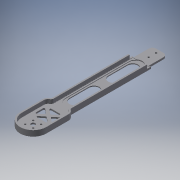
# Autodesk Inventor part: Arm
Saved by Autodesk Inventor 2016 (Build 200138000, 138)
## iProperties
Created: 2015-04-14
Part Number: Arm
Material: Generic
Document SubType Name: Modeling
Designer: Vasanth
Density: 1 g/cm^3
Appearance: Default
Author: Vasanth
Autodesk Inventor part; units mm, degrees
ref_plane "YZ Plane" through (0, 0, 0) normal (1, 0, 0) x (0, 1, 0)
ref_plane "XZ Plane" through (0, 0, 0) normal (0, 1, 0) x (-1, 0, 0)
ref_plane "XY Plane" through (0, 0, 0) normal (0, 0, 1) x (1, 0, 0)
sketch "Sketch1" plane through (0, 0, 0) normal (0, 1, 0) x (-1, 0, 0)
  line L0 (52.0335, 19.2292) -> (51.733, 19.2292)
  line L1 (38.3582, 166.9806) -> (38.3582, 31.0212)
  line L2 (6.6082, 166.9806) -> (6.6082, 31.0212)
  line L3 (38.3582, 31.0212) -> (35.1832, 32.9161)
  line L4 (35.1832, 32.9161) -> (35.1832, 6.5292)
  line L5 (9.7832, 32.9161) -> (9.7832, 6.5292)
  line L6 (16.1332, 0.1792) -> (28.8332, 0.1792)
  line L7 (44.7082, 216.0792) -> (44.7082, 177.9792)
  line L8 (0.2582, 177.9792) -> (0.2582, 216.0792)
  arc A0 (44.7082, 216.0792) -> (0.2582, 216.0792) centre (22.4832, 216.0792) ccw
  arc A1 (39.9457, 169.7303) -> (38.3582, 166.9806) centre (41.5332, 166.9806) ccw
  arc A2 (28.8332, 0.1792) -> (35.1832, 6.5292) centre (28.8332, 6.5292) ccw
  arc A3 (9.7832, 6.5292) -> (16.1332, 0.1792) centre (16.1332, 6.5292) ccw
  arc A4 (39.9457, 169.7303) -> (44.7082, 177.9792) centre (35.1832, 177.9792) ccw
  arc A5 (0.2582, 177.9792) -> (5.0207, 169.7303) centre (9.7832, 177.9792) ccw
  arc A6 (6.6082, 166.9806) -> (5.0207, 169.7303) centre (3.4332, 166.9806) ccw
  line L9 (9.7832, 32.9161) -> (6.6082, 31.0212)
  constraints: 20 end point, 15 tangent, 14 point on circle, 7 centre point, 4 vertical, 3 equal radius, 3 parallel, 1 horizontal
extrude "Extrusion1" add sketch "Sketch1" along normal blind 9.525
sketch "Sketch5" plane through (0, 9.525, 0) normal (0, 1, 0) x (1, 0, 0)
  line L0 (-52.0335, -19.2292) -> (-51.733, -19.2292)
  line L1 (-35.1832, -32.9161) -> (-35.1832, -34.2351)
  line L2 (-9.7832, -32.9161) -> (-9.7832, -34.2351)
  line L3 (-2.7995, -216.0792) -> (-2.7995, -177.9792)
  line L4 (-42.167, -216.0792) -> (-42.167, -177.9792)
  line L5 (-9.1495, -166.9806) -> (-9.1495, -34.2351)
  line L6 (-9.1495, -34.2351) -> (-9.7832, -34.2351)
  line L7 (-35.1832, -34.2351) -> (-35.9386, -34.2351)
  line L8 (-35.1832, -6.5292) -> (-35.1832, -32.9161)
  line L9 (-35.1832, -32.9161) -> (-35.1832, -6.5292) projected
  line L10 (-9.7832, -32.9161) -> (-9.7832, -6.5292)
  arc A0 (-9.7832, -6.5292) -> (-16.1332, -0.1792) centre (-16.1332, -6.5292) ccw
  arc A1 (-28.8332, -0.1792) -> (-35.1832, -6.5292) centre (-28.8332, -6.5292) ccw
  arc A2 (-38.6751, -171.9311) -> (-42.167, -177.9792) centre (-35.1832, -177.9792) ccw
  arc A3 (-2.7995, -177.9792) -> (-6.2914, -171.9311) centre (-9.7832, -177.9792) ccw
  arc A4 (-9.1495, -166.9806) -> (-6.2914, -171.9311) centre (-3.4332, -166.9806) ccw
  arc A5 (-38.6751, -171.9311) -> (-35.9386, -168.1538) centre (-41.5332, -166.9806) ccw
  line L11 (-28.8332, -0.1792) -> (-16.1332, -0.1792)
  arc A6 (-9.7832, -6.5292) -> (-16.1332, -0.1792) centre (-16.1332, -6.5292) ccw projected
  line L12 (-16.1332, -0.1792) -> (-28.8332, -0.1792) projected
  arc A7 (-42.167, -216.0792) -> (-2.7995, -216.0792) centre (-22.4832, -216.0792) ccw
  line L13 (-35.9386, -34.2351) -> (-35.9386, -168.1538)
  line L14 (-38.3582, -166.9806) -> (-38.3582, -31.0212) projected
  constraints: 24 end point, 14 point on circle, 7 centre point, 3 vertical, 2 collinear, 2 parallel, 1 horizontal, 1 point on line, 1 tangent
extrude "Extrusion2" cut sketch "Sketch5" against normal blind 6.35
sketch "Sketch6" plane through (0, 9.525, 0) normal (0, 1, 0) x (1, 0, 0)
  circle A0 centre (-22.4832, -19.2292) radius 1.5001
  circle A1 centre (-22.4832, -6.5292) radius 1.5001
  line L0 (-13.5932, -145.3906) -> (-13.5932, -112.3706)
  line L1 (-31.3732, -145.3906) -> (-31.3732, -112.3706)
  line L2 (-31.3732, -79.3506) -> (-31.3732, -46.3306)
  line L3 (-13.5932, -79.3506) -> (-13.5932, -46.3306)
  arc A2 (-13.5932, -112.3706) -> (-31.3732, -112.3706) centre (-22.4832, -112.3706) ccw
  arc A3 (-31.3732, -145.3906) -> (-13.5932, -145.3906) centre (-22.4832, -145.3906) ccw
  arc A4 (-31.3732, -79.3506) -> (-13.5932, -79.3506) centre (-22.4832, -79.3506) ccw
  arc A5 (-13.5932, -46.3306) -> (-31.3732, -46.3306) centre (-22.4832, -46.3306) ccw
  line L4 (-149.0334, -127.8705) -> (-176.2084, -108.4598)
  line L5 (-109.1652, -138.2049) -> (-81.9901, -157.6157)
  line L6 (-123.9321, -113.1036) -> (-104.5213, -85.9286)
  line L7 (-109.6885, -190.1877) -> (-148.51, -190.1877)
  line L8 (-109.6885, -75.8877) -> (-148.51, -75.8877)
  arc A6 (-148.51, -75.8877) -> (-153.6772, -85.9286) centre (-148.51, -82.2377) ccw
  circle A7 centre (-82.019, -85.9575) radius 1.5001
  circle A8 centre (-176.1795, -180.118) radius 1.5001
  circle A9 centre (-176.1795, -85.9575) radius 1.5001
  circle A10 centre (-151.5993, -155.5378) radius 1.5001
  circle A11 centre (-106.5992, -155.5378) radius 1.5001
  circle A12 centre (-106.5992, -110.5377) radius 1.5001
  circle A13 centre (-151.5993, -110.5377) radius 1.5001
  circle A14 centre (-16.8264, -221.736) radius 1.5001
  circle A15 centre (-29.2008, -222.7967) radius 1.5001
  circle A16 centre (-15.7656, -209.3616) radius 1.5001
  line L9 (-149.0334, -138.2049) -> (-176.2084, -157.6157)
  line L10 (-134.2665, -152.9718) -> (-153.6772, -180.1469)
  line L11 (-109.1652, -127.8705) -> (-81.9901, -108.4598)
  line L12 (-134.2665, -113.1036) -> (-153.6772, -85.9286)
  line L13 (-186.2493, -113.627) -> (-186.2493, -152.4485)
  line L14 (-71.9493, -152.4485) -> (-71.9493, -113.627)
  arc A17 (-104.5213, -85.9286) -> (-109.6885, -75.8877) centre (-109.6885, -82.2377) ccw
  arc A18 (-134.2665, -113.1036) -> (-123.9321, -113.1036) centre (-129.0993, -109.4128) ccw
  arc A19 (-149.0334, -138.2049) -> (-149.0334, -127.8705) centre (-152.7242, -133.0377) ccw
  arc A20 (-186.2493, -152.4485) -> (-176.2084, -157.6157) centre (-179.8993, -152.4485) ccw
  arc A21 (-176.2084, -108.4598) -> (-186.2493, -113.627) centre (-179.8993, -113.627) ccw
  arc A22 (-153.6772, -180.1469) -> (-148.51, -190.1877) centre (-148.51, -183.8377) ccw
  arc A23 (-123.9321, -152.9718) -> (-134.2665, -152.9718) centre (-129.0993, -156.6627) ccw
  arc A24 (-81.9901, -157.6157) -> (-71.9493, -152.4485) centre (-78.2993, -152.4485) ccw
  arc A25 (-71.9493, -113.627) -> (-81.9901, -108.4598) centre (-78.2993, -113.627) ccw
  arc A26 (-109.1652, -127.8705) -> (-109.1652, -138.2049) centre (-105.4743, -133.0377) ccw
  arc A27 (-127.8075, -223.1112) -> (-130.3911, -223.1112) centre (-129.0993, -224.034) ccw
  line L15 (-134.0828, -216.8359) -> (-140.8766, -211.9832)
  line L16 (-134.0828, -219.4195) -> (-140.8766, -224.2722)
  line L17 (-127.8075, -223.1112) -> (-122.9548, -229.905)
  line L18 (-130.3911, -223.1112) -> (-135.2438, -229.905)
  line L19 (-124.1158, -219.4195) -> (-117.322, -224.2722)
  line L20 (-124.1158, -216.8359) -> (-117.322, -211.9832)
  line L21 (-127.8075, -213.1442) -> (-122.9548, -206.3504)
  line L22 (-130.3911, -213.1442) -> (-135.2437, -206.3504)
  arc A28 (-130.3911, -213.1442) -> (-127.8075, -213.1442) centre (-129.0993, -212.2215) ccw
  arc A29 (-134.0828, -219.4195) -> (-134.0828, -216.8359) centre (-135.0055, -218.1277) ccw
  arc A30 (-124.1158, -216.8359) -> (-124.1158, -219.4195) centre (-123.193, -218.1277) ccw
  line L23 (-117.322, -224.2722) -> (-108.7122, -230.3009)
  line L24 (-117.322, -211.9832) -> (-108.7122, -205.9546)
  line L25 (-135.2438, -229.905) -> (-137.004, -232.4188)
  line L26 (-122.9548, -229.905) -> (-121.1946, -232.4188)
  line L27 (-123.2752, -236.4157) -> (-134.9233, -236.4157)
  line L28 (-123.24, -199.8397) -> (-134.9586, -199.8397)
  line L29 (-153.4832, -207.9142) -> (-153.4832, -228.3413)
  line L30 (-104.7153, -228.2202) -> (-104.7153, -208.0352)
  line L31 (-140.8766, -211.9832) -> (-149.4669, -205.8473)
  line L32 (-140.8766, -224.2722) -> (-149.4669, -230.4082)
  line L33 (-122.9548, -206.3504) -> (-121.1731, -203.8561)
  line L34 (-135.2437, -206.3504) -> (-137.0254, -203.8561)
  arc A31 (-108.7122, -230.3009) -> (-104.7153, -228.2202) centre (-107.2553, -228.2202) ccw
  arc A32 (-104.7153, -208.0352) -> (-108.7122, -205.9546) centre (-107.2553, -208.0352) ccw
  arc A33 (-121.1731, -203.8561) -> (-123.24, -199.8397) centre (-123.24, -202.3797) ccw
  arc A34 (-134.9586, -199.8397) -> (-137.0254, -203.8561) centre (-134.9586, -202.3797) ccw
  arc A35 (-149.4669, -205.8473) -> (-153.4832, -207.9142) centre (-150.9432, -207.9142) ccw
  arc A36 (-153.4832, -228.3413) -> (-149.4669, -230.4082) centre (-150.9432, -228.3413) ccw
  arc A37 (-137.004, -232.4188) -> (-134.9233, -236.4157) centre (-134.9233, -233.8757) ccw
  arc A38 (-123.2752, -236.4157) -> (-121.1946, -232.4188) centre (-123.2752, -233.8757) ccw
  arc A39 (-109.6885, -190.1877) -> (-104.5213, -180.1469) centre (-109.6885, -183.8377) ccw
  line L35 (-123.9321, -152.9718) -> (-104.5213, -180.1469)
  circle A40 centre (-82.019, -180.118) radius 1.5001
  circle A41 centre (-22.4832, -216.0792) radius 3.5001
  circle A42 centre (-28.1401, -210.4223) radius 1.5001
  arc A43 (-92.1218, -170.0152) -> (-89.8767, -172.2603) centre (-90.9993, -171.1377) ccw
  arc A44 (-82.019, -169.0055) -> (-82.019, -165.8305) centre (-82.019, -167.418) ccw
  arc A45 (-82.019, -169.0055) -> (-89.8767, -172.2603) centre (-82.019, -180.118) ccw
  arc A46 (-82.019, -165.8305) -> (-92.1218, -170.0152) centre (-82.019, -180.118) ccw
  arc A47 (-82.019, -100.245) -> (-82.019, -97.07) centre (-82.019, -98.6575) ccw
  arc A48 (-92.1218, -96.0603) -> (-82.019, -100.245) centre (-82.019, -85.9575) ccw
  arc A49 (-89.8767, -93.8152) -> (-82.019, -97.07) centre (-82.019, -85.9575) ccw
  arc A50 (-89.8767, -93.8152) -> (-92.1218, -96.0603) centre (-90.9993, -94.9377) ccw
  arc A51 (-176.1795, -165.8305) -> (-176.1795, -169.0055) centre (-176.1795, -167.418) ccw
  arc A52 (-166.0767, -170.0152) -> (-176.1795, -165.8305) centre (-176.1795, -180.118) ccw
  arc A53 (-168.3218, -172.2603) -> (-176.1795, -169.0055) centre (-176.1795, -180.118) ccw
  arc A54 (-168.3218, -172.2603) -> (-166.0767, -170.0152) centre (-167.1993, -171.1377) ccw
  arc A55 (-176.1795, -97.07) -> (-176.1795, -100.245) centre (-176.1795, -98.6575) ccw
  arc A56 (-176.1795, -100.245) -> (-166.0767, -96.0603) centre (-176.1795, -85.9575) ccw
  arc A57 (-176.1795, -97.07) -> (-168.3218, -93.8152) centre (-176.1795, -85.9575) ccw
  arc A58 (-166.0767, -96.0603) -> (-168.3218, -93.8152) centre (-167.1993, -94.9377) ccw
  arc A59 (-15.4908, -202.4266) -> (-14.4897, -199.6071) centre (-15.4908, -200.8391) ccw
  arc A60 (-30.4768, -199.6071) -> (-29.4757, -202.4266) centre (-29.4757, -200.8391) ccw
  arc A61 (-21.4822, -193.9257) -> (-23.4843, -193.9257) centre (-22.4832, -195.1578) ccw
  arc A62 (-17.1906, -188.8121) -> (-17.1906, -191.2762) centre (-16.1895, -190.0442) ccw
  arc A63 (-7.2432, -184.0651) -> (-9.8318, -182.833) centre (-8.8307, -184.0651) ccw
  arc A64 (-9.8318, -197.2553) -> (-7.2432, -196.0232) centre (-8.8307, -196.0232) ccw
  arc A65 (-14.4897, -180.4812) -> (-15.4908, -177.6617) centre (-15.4908, -179.2492) ccw
  arc A66 (-29.4757, -177.6617) -> (-30.4768, -180.4812) centre (-29.4757, -179.2492) ccw
  arc A67 (-23.4843, -186.1626) -> (-21.4822, -186.1626) centre (-22.4832, -184.9305) ccw
  arc A68 (-27.7758, -191.2762) -> (-27.7758, -188.8121) centre (-28.7769, -190.0442) ccw
  arc A69 (-37.7232, -196.0232) -> (-35.1347, -197.2553) centre (-36.1357, -196.0232) ccw
  arc A70 (-35.1347, -182.833) -> (-37.7232, -184.0651) centre (-36.1357, -184.0651) ccw
  line L36 (-15.4908, -202.4266) -> (-29.4757, -202.4266)
  line L37 (-14.4897, -199.6071) -> (-21.4822, -193.9257)
  line L38 (-23.4843, -193.9257) -> (-30.4768, -199.6071)
  line L39 (-35.1347, -197.2553) -> (-27.7758, -191.2762)
  line L40 (-27.7758, -188.8121) -> (-35.1347, -182.833)
  line L41 (-37.7232, -184.0651) -> (-37.7232, -196.0232)
  line L42 (-30.4768, -180.4812) -> (-23.4843, -186.1626)
  line L43 (-21.4822, -186.1626) -> (-14.4897, -180.4812)
  line L44 (-15.4908, -177.6617) -> (-29.4757, -177.6617)
  line L45 (-7.2432, -196.0232) -> (-7.2432, -184.0651)
  line L46 (-9.8318, -182.833) -> (-17.1906, -188.8121)
  line L47 (-17.1906, -191.2762) -> (-9.8318, -197.2553)
  point P0 (0, 0)
  constraints: 112 point on circle, 99 tangent, 96 end point, 71 centre point, 49 equal radius, 10 parallel, 10 perpendicular, 8 concentric, 2 collinear
extrude "Extrusion3" cut sketch "Sketch6" against normal blind 25.4
sketch "Sketch7" plane through (0, 9.525, 0) normal (0, 1, 0) x (1, 0, 0)
  line L0 (-52.0335, -19.2292) -> (-51.733, -19.2292)
  line L1 (0, -16.7662) -> (-44.6659, -16.7662)
  line L2 (0, -38.112) -> (-44.6659, -38.112)
  line L3 (0, -38.112) -> (0, -16.7662)
  line L4 (-44.6659, -16.7662) -> (-44.6659, -38.112)
  point P0 (0, 0)
  constraints: 10 end point
extrude "Extrusion4" cut sketch "Sketch7" against normal blind 6.35
sketch "Sketch9" plane through (0, 9.525, 0) normal (0, 1, 0) x (1, 0, 0)
  arc A0 (-6.6082, -166.9806) -> (-5.0207, -169.7303) centre (-3.4332, -166.9806) ccw
  spline S0 degree 2 poles (-33.6688, -150.3436) (-33.6688, -161.5196) (-22.5213, -161.5196) (-11.3739, -161.5196) (-11.3739, -150.3436) knots 0 0 0 1 1 2 2 2 weights 1 0.707107 1 0.707107 1
  line L0 (-33.6688, -150.3436) -> (-33.6688, -161.5196) construction
  line L1 (-33.6688, -161.5196) -> (-22.5213, -161.5196) construction
  line L2 (-22.5213, -161.5196) -> (-11.3739, -161.5196) construction
  line L3 (-11.3739, -161.5196) -> (-11.3739, -150.3436) construction
  arc A1 (-11.3739, -41.3776) -> (-33.6688, -41.3776) centre (-22.5213, -41.3776) ccw
  line L4 (-11.3739, -150.3436) -> (-11.3739, -41.3776)
  line L5 (-33.6688, -41.3776) -> (-33.6688, -150.3436)
  point P0 (0, 0)
  constraints: 4 end point, 4 point on circle, 2 centre point, 1 parallel, 1 vertical, 3 other
extrude "Extrusion6" cut sketch "Sketch9" against normal blind 8.001
sketch "Sketch10" plane through (0, 3.175, 0) normal (0, 1, 0) x (1, 0, 0)
  line L0 (-52.0335, -19.2292) -> (-51.733, -19.2292)
  arc A0 (-38.6751, -171.9311) -> (-35.817, -166.9806) centre (-41.5332, -166.9806) ccw
  arc A1 (-38.6751, -171.9311) -> (-42.167, -177.9792) centre (-35.1832, -177.9792) ccw
  line L1 (-42.167, -177.9792) -> (-42.167, -216.0792)
  arc A2 (-42.167, -216.0792) -> (-2.7995, -216.0792) centre (-22.4832, -216.0792) ccw
  line L2 (-2.7995, -216.0792) -> (-2.7995, -177.9792)
  arc A3 (-2.7995, -177.9792) -> (-6.2914, -171.9311) centre (-9.7832, -177.9792) ccw
  arc A4 (-9.1495, -166.9806) -> (-6.2914, -171.9311) centre (-3.4332, -166.9806) ccw
  line L3 (-9.1495, -166.9806) -> (-9.1495, -34.2351)
  line L4 (-35.817, -34.2351) -> (-35.817, -166.9806)
  line L5 (-35.1832, -32.9161) -> (-35.817, -32.9161)
  line L6 (-9.7832, -32.9161) -> (-9.1495, -32.9161)
  line L7 (-9.1495, -34.2351) -> (-9.1495, -32.9161)
  line L8 (-35.817, -34.2351) -> (-35.817, -32.9161)
  line L9 (-35.1832, -32.9161) -> (-9.1495, -32.9161)
  point P0 (-9.1495, -166.9806)
  point P1 (-41.5332, -166.9806)
  point P2 (-3.4332, -166.9806)
  constraints: 20 end point, 10 point on circle, 6 tangent, 5 centre point, 2 equal radius, 2 perpendicular
extrude "Extrusion7" cut sketch "Sketch10" against normal blind 0.635
thread "Thread1" size "5-40 UNC" class "2B" standard "ANSI Unified Screw Threads" full length
thread "Thread2" size "5-40 UNC" class "2B" standard "ANSI Unified Screw Threads" full length
body "Solid1"
